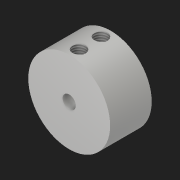
# Autodesk Inventor part: AA050
Saved by Autodesk Inventor 2017 SP1 (Build 210196100, 196)
## iProperties
Created: 2018-02-16
Part Number: AA050
Material: Aluminum 6061
Document SubType Name: Modeling
Designer: Zach
Density: 2.7 g/cm^3
Appearance: Aluminum - Flat
Author: Zach
Autodesk Inventor part; units mm, degrees
ref_plane "YZ Plane" through (0, 0, 0) normal (1, 0, 0) x (0, 1, 0)
ref_plane "XZ Plane" through (0, 0, 0) normal (0, 1, 0) x (-1, 0, 0)
ref_plane "XY Plane" through (0, 0, 0) normal (0, 0, 1) x (1, 0, 0)
sketch "Sketch1" plane through (0, 0, 0) normal (0, 0, 1) x (1, 0, 0)
  circle A0 centre (0, 0) radius 12.5
  circle A1 centre (0, 0) radius 2
  dimension "d1" = 4
  dimension "d32" = 25
  constraints: 2 centre point, 2 coincident
  measures "d1" diameter of A1
  measures "d32" diameter of A0
extrude "Extrusion1" add sketch "Sketch1" along normal blind 12.7
sketch "Sketch8" plane through (0, 0, 0) normal (0, 1, 0) x (-1, 0, 0)
  circle A0 centre (0, 3) radius 2
  circle A1 centre (0, 9.7) radius 2
  line L0 (2, 0) -> (-2, 0) projected
  line L1 (-2, 12.7) -> (2, 12.7) projected
  point P0 (0, 0)
  point P1 (0, 0)
  dimension "d33" = 4
  dimension "d34" = 4
  dimension "d35" = 3
  dimension "d36" = 3
  constraints: 2 centre point, 2 vertical alignment, 1 midpoint
  measures "d33" diameter of A0
  measures "d34" diameter of A1
  measures "d35" distance from line of L0 A0.centre
  measures "d36" distance from line of L1 A1.centre
extrude "Extrusion6" cut sketch "Sketch8" along normal through all
sketch "Sketch9" plane through (0, 0, 0) normal (0, 0, -1) x (-1, 0, 0)
  circle A0 centre (0, 0) radius 3
  dimension "d39" = 6
  constraints: 1 centre point, 1 coincident
  measures "d39" diameter of A0
extrude "Extrusion7" cut sketch "Sketch9" against normal blind 6.35
thread "Thread1" size "M4x0.7" class "6H" standard "ANSI Metric M Profile" full length
thread "Thread2" size "M4x0.7" class "6H" standard "ANSI Metric M Profile" full length
body "Solid1"
